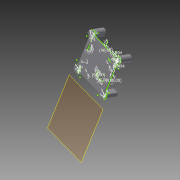
# Autodesk Inventor part: Ceiling
Saved by Autodesk Inventor 2015 (Build 190159000, 159)
## iProperties
Created: 2015-06-02
Part Number: Ceiling
Material: Generic
Document SubType Name: Modeling
Designer: Vu
Density: 1 g/cm^3
Appearance: Default
Author: Vu
Autodesk Inventor part; units mm, degrees
ref_plane "YZ Plane" through (0, 0, 0) normal (1, 0, 0) x (0, 1, 0)
ref_plane "XZ Plane" through (0, 0, 0) normal (0, 1, 0) x (-1, 0, 0)
ref_plane "XY Plane" through (0, 0, 0) normal (0, 0, 1) x (1, 0, 0)
ref_plane "Work Plane1" through (219.9513, -256.0439, -597.7148) normal (-0.0970089, -0.9550916, 0.2799809) x (-0.2030452, -0.2564002, -0.9450035)
sketch "Sketch3" plane through (219.9513, -256.0439, -597.7148) normal (-0.0970089, -0.9550916, 0.2799809) x (-0.2030452, -0.2564002, -0.9450035)
  line L0 (-0.0023, 59.9989) -> (-40.0023, 59.9989)
  line L1 (-0.0023, 59.9989) -> (39.9977, 59.9989) construction
  line L2 (-60.0163, -0.0152) -> (-60.0163, 39.9848)
  line L3 (-60.0163, -0.0152) -> (-20.0163, -0.0152) construction
  line L4 (-60.0163, -0.0152) -> (-0.0023, -0.0152)
  line L5 (-0.0023, -0.0152) -> (-0.0023, 59.9989)
  arc A0 (-49.9687, 64.958) -> (-40.0023, 59.9989) centre (-40.0023, 72.4933) ccw
  arc A1 (-60.0163, 39.9848) -> (-64.9755, 49.9513) centre (-72.5108, 39.9848) ccw
  arc A2 (-49.9687, 64.958) -> (-64.9755, 49.9513) centre (-58.5144, 58.4969) ccw
  line L6 (-40.0023, 59.9989) -> (-40.0023, 59.4989)
  line L7 (-60.0163, 39.9848) -> (-59.5163, 39.9848)
  arc A3 (-59.5163, 39.9848) -> (-40.0023, 59.4989) centre (-59.5163, 59.4989) ccw
  line L8 (-60.0163, -0.0152) -> (-80.0163, -0.0152)
  line L9 (-60.0163, -40.0152) -> (-59.5163, -40.0152)
  arc A4 (-64.9755, -49.9816) -> (-60.0163, -40.0152) centre (-72.5108, -40.0152) ccw
  line L10 (-60.0163, -0.0152) -> (-60.0163, -40.0152)
  arc A5 (-64.9755, -49.9816) -> (-49.9687, -64.9884) centre (-58.5144, -58.5273) ccw
  arc A6 (-40.0023, -60.0292) -> (-49.9687, -64.9884) centre (-40.0023, -72.5237) ccw
  arc A7 (-40.0023, -59.5292) -> (-59.5163, -40.0152) centre (-59.5163, -59.5292) ccw
  line L11 (-40.0023, -60.0292) -> (-40.0023, -59.5292)
  line L12 (-0.0023, -60.0292) -> (-40.0023, -60.0292)
  line L13 (-0.0023, -0.0152) -> (-0.0023, -60.0292)
  line L14 (-0.0023, 59.9989) -> (-40.0023, 59.9989) construction
  line L15 (-0.0023, 59.9989) -> (39.9977, 59.9989)
  line L16 (60.0118, -0.0152) -> (60.0118, 39.9848)
  line L17 (60.0118, 39.9848) -> (59.5118, 39.9848)
  arc A8 (64.9709, 49.9513) -> (60.0118, 39.9848) centre (72.5063, 39.9848) ccw
  line L18 (60.0118, -0.0152) -> (20.0118, -0.0152) construction
  arc A9 (64.9709, 49.9513) -> (49.9642, 64.958) centre (58.5098, 58.4969) ccw
  arc A10 (39.9977, 59.4989) -> (59.5118, 39.9848) centre (59.5118, 59.4989) ccw
  line L19 (39.9977, 59.9989) -> (39.9977, 59.4989)
  arc A11 (39.9977, 59.9989) -> (49.9642, 64.958) centre (39.9977, 72.4933) ccw
  line L20 (60.0118, -0.0152) -> (-0.0023, -0.0152)
  line L21 (60.0118, -40.0152) -> (59.5118, -40.0152)
  line L22 (60.0118, -0.0152) -> (60.0118, -40.0152)
  arc A12 (60.0118, -40.0152) -> (64.9709, -49.9816) centre (72.5063, -40.0152) ccw
  arc A13 (59.5118, -40.0152) -> (39.9977, -59.5292) centre (59.5118, -59.5292) ccw
  arc A14 (49.9642, -64.9884) -> (64.9709, -49.9816) centre (58.5098, -58.5273) ccw
  line L23 (39.9977, -60.0292) -> (39.9977, -59.5292)
  arc A15 (49.9642, -64.9884) -> (39.9977, -60.0292) centre (39.9977, -72.5237) ccw
  line L24 (-0.0023, -60.0292) -> (39.9977, -60.0292)
  line L25 (10, 10) -> (30, 10)
  line L26 (30, 10) -> (30, 40)
  line L27 (30, 40) -> (10, 40)
  line L28 (10, 40) -> (10, 10)
  line L29 (-30, -52.5) -> (-10, -52.5)
  line L30 (-10, -52.5) -> (-10, -45.5)
  line L31 (-10, -45.5) -> (-30, -45.5)
  line L32 (-30, -45.5) -> (-30, -52.5)
  ellipse E0 centre (-40.0023, 32.8682) end of major axis (-38.2648, 42.8976) minor radius 3.285
  circle A16 centre (12, 6) radius 1.5
  circle A17 centre (18, 6) radius 1.5
  circle A18 centre (24, 6) radius 1.5
  circle A19 centre (45, -22) radius 1.5
  circle A20 centre (27, -45) radius 1.5
  circle A21 centre (-25, 35) radius 1.5
  circle A22 centre (-52.5, 52.5) radius 2
  circle A23 centre (-55.5, 62.5) radius 2
  circle A24 centre (-62.5, 55.5) radius 2
  circle A25 centre (-62.5, -55.5303) radius 2
  circle A26 centre (-55.5, -62.5303) radius 2
  circle A27 centre (-52.5, -52.5303) radius 2
  circle A28 centre (52.4955, -52.5303) radius 2
  circle A29 centre (55.4955, -62.5303) radius 2
  circle A30 centre (62.4955, -55.5303) radius 2
  circle A31 centre (52.4955, 52.5) radius 2
  circle A32 centre (55.4955, 62.5) radius 2
  circle A33 centre (62.4955, 55.5) radius 2
  line L33 (52.4955, 52.5) -> (57.4955, 52.5) construction
  line L34 (48.96, 48.9645) -> (49.9642, 64.958)
  line L35 (48.96, 48.9645) -> (64.9709, 49.9513)
  line L36 (52.4955, -52.5303) -> (57.4955, -52.5303) construction
  line L37 (64.9709, -49.9816) -> (48.96, -48.9948)
  line L38 (48.96, -48.9948) -> (49.9642, -64.9884)
  line L39 (-52.5, -52.5303) -> (-47.5, -52.5303) construction
  line L40 (-49.9687, -64.9884) -> (-48.9645, -48.9948)
  line L41 (-64.9755, -49.9816) -> (-48.9645, -48.9948)
  line L42 (-52.5, 52.5) -> (-48.9645, 48.9645)
  line L43 (-52.5, 52.5) -> (-47.5, 52.5) construction
  line L44 (-48.9645, 48.9645) -> (-64.9755, 49.9513)
  line L45 (-48.9645, 48.9645) -> (-49.9687, 64.958)
  circle A34 centre (-23, -40) radius 1.5
  dimension "d14" = 40
  dimension "d15" = 180
  dimension "d16" = 40
  dimension "d17" = 90
  dimension "d18" = 12.4944
  dimension "d19" = 12.4944
  dimension "d20" = 0.5
  dimension "d21" = 0.5
  dimension "d22" = 20
  dimension "d24" = 20
  dimension "d25" = 30
  dimension "d26" = 90
  dimension "d27" = 90
  dimension "d28" = 20
  dimension "d29" = 7
  dimension "d30" = 3
  dimension "d31" = 3
  dimension "d32" = 3
  dimension "d33" = 3
  dimension "d34" = 3
  dimension "d35" = 3
  dimension "d36" = 4
  dimension "d37" = 4
  dimension "d38" = 4
  dimension "d39" = 4
  dimension "d40" = 4
  dimension "d41" = 4
  dimension "d42" = 4
  dimension "d43" = 4
  dimension "d44" = 4
  dimension "d45" = 4
  dimension "d46" = 4
  dimension "d47" = 4
  dimension "d54" = 5
  dimension "d56" = 5
  dimension "d58" = 5
  dimension "d59" = 45
  dimension "d62" = 3
  constraints: 92 end point, 43 symmetric about line, 35 centre point, 32 point on circle, 12 coincident, 12 horizontal, 6 tangent, 4 perpendicular, 3 equal length, 2 parallel, 2 vertical, 14 other
  measures "d14" distance of L0.start L0.end
  measures "d15" angle of L0 L1
  measures "d16" distance of L2.start L2.end
  measures "d17" angle of L3 L2
  measures "d18" radius of A0
  measures "d19" radius of A1
  measures "d20" distance of L0.end L6.end
  measures "d21" distance of L2.end L7.end
  measures "d22" distance of L2.start L8.end
  measures "d24" distance of L25.start L25.end
  measures "d25" distance of L25.end L26.end
  measures "d26" angle of L26 L25
  measures "d27" angle of L27 L26
  measures "d28" distance of L31.end L30.end
  measures "d29" distance of L30.end L29.end
  measures "d30" diameter of A16
  measures "d31" diameter of A17
  measures "d32" diameter of A18
  measures "d33" diameter of A19
  measures "d34" diameter of A20
  measures "d35" diameter of A21
  measures "d36" diameter of A22
  measures "d37" diameter of A23
  measures "d38" diameter of A24
  measures "d39" diameter of A25
  measures "d40" diameter of A26
  measures "d41" diameter of A27
  measures "d42" diameter of A28
  measures "d43" diameter of A29
  measures "d44" diameter of A30
  measures "d45" diameter of A31
  measures "d46" diameter of A32
  measures "d47" diameter of A33
  measures "d54" distance of L36.start L37.end
  measures "d56" distance of L39.start L40.end
  measures "d58" distance of L42.start L42.end
  measures "d59" angle of L42 L43
  measures "d62" diameter of A34
extrude "Extrusion1" add sketch "Sketch3" along normal blind 4 contours L5 L4 L2 L7 A3 L6 L0 | L15 L19 A10 L17 L16 L20 L5 | L6 A3 L7 A1 L44 L45 A0 | L13 L12 L11 A7 L9 L10 L4 | L20 L22 L21 A13 L23 L24 L13 | A11 L34 L35 A8 L17 A10 L19 | L45 L44 A2 | A9 L35 L34 | L9 A7 L11 A6 L40 L41 A4 | L23 A13 L21 A12 L37 L38 A15 | L41 L40 A5 | L38 L37 A14 | A34
extrude "Extrusion3" add sketch "Sketch3" against normal blind 40 contours L45 L44 A2 | A9 L35 L34 | L41 L40 A5 | L38 L37 A14
extrude "Extrusion4" cut sketch "Sketch3" along normal blind 4 contours A34
body "Solid1"
